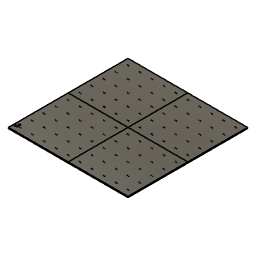
Base Plate (Autodesk Fusion 360 design; units mm, degrees)
Autodesk Fusion 360 part; units mm, degrees
note: some values were not read from the file. Chosen so that the rebuilt part matches the saved one: which face or edge a step refers to.
box "BoxPrimitive1" add length 175 width 175 height 3 placed x (0, 1, 0) y (-1, 0, 0) z (0, 0, 1) at (175, 0, 0) makes body 1
sketch "Sketch2" plane through (0, 0, 3) normal (0, 0, 1) x (-1, 0, 0)
  line L0 (-175, -175) -> (0, -175)
  line L1 (0, -175) -> (0, 0)
  line L2 (0, 0) -> (-175, 0)
  line L3 (-175, 0) -> (-175, -175)
  line L4 (0, 0) -> (-15.5, 0)
  line L5 (-15.5, 0) -> (-15.5, -17.5)
  line L6 (-15.5, -17.5) -> (0, -17.5)
  line L7 (0, -17.5) -> (0, 0)
  line L8 (-15.5, -17.5) -> (-19.5, -17.5)
  circle A0 centre (-19.5, -17.5) radius 0.425
  circle A1 centre (-15.5, -17.5) radius 0.425
  circle A2 centre (-50.5, -17.5) radius 0.425
  circle A3 centre (-54.5, -17.5) radius 0.425
  circle A4 centre (-85.5, -17.5) radius 0.425
  circle A5 centre (-89.5, -17.5) radius 0.425
  circle A6 centre (-120.5, -17.5) radius 0.425
  circle A7 centre (-124.5, -17.5) radius 0.425
  circle A8 centre (-155.5, -17.5) radius 0.425
  circle A9 centre (-159.5, -17.5) radius 0.425
  circle A10 centre (-15.5, -52.5) radius 0.425
  circle A11 centre (-19.5, -52.5) radius 0.425
  circle A12 centre (-50.5, -52.5) radius 0.425
  circle A13 centre (-54.5, -52.5) radius 0.425
  circle A14 centre (-85.5, -52.5) radius 0.425
  circle A15 centre (-89.5, -52.5) radius 0.425
  circle A16 centre (-120.5, -52.5) radius 0.425
  circle A17 centre (-124.5, -52.5) radius 0.425
  circle A18 centre (-155.5, -52.5) radius 0.425
  circle A19 centre (-159.5, -52.5) radius 0.425
  circle A20 centre (-15.5, -87.5) radius 0.425
  circle A21 centre (-19.5, -87.5) radius 0.425
  circle A22 centre (-50.5, -87.5) radius 0.425
  circle A23 centre (-54.5, -87.5) radius 0.425
  circle A24 centre (-85.5, -87.5) radius 0.425
  circle A25 centre (-89.5, -87.5) radius 0.425
  circle A26 centre (-120.5, -87.5) radius 0.425
  circle A27 centre (-124.5, -87.5) radius 0.425
  circle A28 centre (-155.5, -87.5) radius 0.425
  circle A29 centre (-159.5, -87.5) radius 0.425
  circle A30 centre (-15.5, -122.5) radius 0.425
  circle A31 centre (-19.5, -122.5) radius 0.425
  circle A32 centre (-50.5, -122.5) radius 0.425
  circle A33 centre (-54.5, -122.5) radius 0.425
  circle A34 centre (-85.5, -122.5) radius 0.425
  circle A35 centre (-89.5, -122.5) radius 0.425
  circle A36 centre (-120.5, -122.5) radius 0.425
  circle A37 centre (-124.5, -122.5) radius 0.425
  circle A38 centre (-155.5, -122.5) radius 0.425
  circle A39 centre (-159.5, -122.5) radius 0.425
  circle A40 centre (-15.5, -157.5) radius 0.425
  circle A41 centre (-19.5, -157.5) radius 0.425
  circle A42 centre (-50.5, -157.5) radius 0.425
  circle A43 centre (-54.5, -157.5) radius 0.425
  circle A44 centre (-85.5, -157.5) radius 0.425
  circle A45 centre (-89.5, -157.5) radius 0.425
  circle A46 centre (-120.5, -157.5) radius 0.425
  circle A47 centre (-124.5, -157.5) radius 0.425
  circle A48 centre (-155.5, -157.5) radius 0.425
  circle A49 centre (-159.5, -157.5) radius 0.425
  dimension "d6" = 15.5
  dimension "d7" = 17.5
  dimension "d8" = 4
  dimension "d9" = 0.85
  dimension "d10" = 0.85
  dimension "d13" = -35
  dimension "d14" = -35
  constraint horizontal L4
  constraint vertical L5
  constraint horizontal L6
  constraint vertical L7
  constraint coincident L1.end L2.start
  constraint perpendicular L5 L8
  constraint coincident L8.end A0.centre
  constraint coincident L5.end L6.start
  measures "d6" distance of L1.end L4.end
  measures "d7" distance of L1.end L6.end
  measures "d8" distance of L5.end L8.end
  measures "d9" diameter of A0
  measures "d10" diameter of A1
hole "Hole1" at (89.5, 157.5, 3) at (159.5, 157.5, 3) at (85.5, 157.5, 3) at (19.5, 157.5, 3) at (50.5, 157.5, 3) at (54.5, 157.5, 3) at (120.5, 157.5, 3) at (124.5, 157.5, 3) at (155.5, 157.5, 3) at (15.5, 157.5, 3) at (89.5, 122.5, 3) at (19.5, 52.5, 3) at (120.5, 87.5, 3) at (15.5, 52.5, 3) at (19.5, 87.5, 3) at (120.5, 122.5, 3) at (50.5, 87.5, 3) at (124.5, 87.5, 3) at (15.5, 122.5, 3) at (89.5, 52.5, 3) at (155.5, 52.5, 3) at (124.5, 122.5, 3) at (50.5, 52.5, 3) at (124.5, 52.5, 3) at (120.5, 52.5, 3) at (19.5, 122.5, 3) at (155.5, 87.5, 3) at (89.5, 87.5, 3) at (159.5, 52.5, 3) at (159.5, 122.5, 3) at (85.5, 87.5, 3) at (54.5, 122.5, 3) at (15.5, 87.5, 3) at (50.5, 122.5, 3) at (155.5, 122.5, 3) at (54.5, 52.5, 3) at (85.5, 52.5, 3) at (159.5, 87.5, 3) at (85.5, 122.5, 3) at (54.5, 87.5, 3) at (85.5, 17.5, 3) at (50.5, 17.5, 3) at (120.5, 17.5, 3) at (159.5, 17.5, 3) at (155.5, 17.5, 3) at (124.5, 17.5, 3) at (54.5, 17.5, 3) at (89.5, 17.5, 3) at (19.5, 17.5, 3) at (19.5, 17.5, 3) at (15.5, 17.5, 3) at (15.5, 17.5, 3) direction (0, 0, -1) diameter 1.1 depth 2.4 tip angle 180 countersink diameter 1.5 countersink angle 40 bodies 1
mirror "Mirror1" about plane through (175, 0, 0) normal (1, 0, 0) of bodies 1 makes body 2
mirror "Mirror2" about plane through (175, 0, 0) normal (0, -1, 0) of bodies 1 2 makes body 3 at (58.3333, -58.3333, 0) makes body 4 at (291.6667, -58.3333, 0)
sketch "Sketch3" plane through (0, 0, 3) normal (0, 0, 1) x (-1, 0, 0)
  circle A0 centre (-54.5, 17.5) radius 0.75
  circle A1 centre (-155.5, 17.5) radius 0.75
  circle A2 centre (-120.5, 17.5) radius 0.75
  circle A3 centre (-85.5, 17.5) radius 0.75
  circle A4 centre (-85.5, 122.5) radius 0.75
  circle A5 centre (-85.5, 52.5) radius 0.75
  circle A6 centre (-155.5, 122.5) radius 0.75
  circle A7 centre (-15.5, 87.5) radius 0.75
  circle A8 centre (-85.5, 87.5) radius 0.75
  circle A9 centre (-159.5, 52.5) radius 0.75
  circle A10 centre (-155.5, 87.5) radius 0.75
  circle A11 centre (-120.5, 52.5) radius 0.75
  circle A12 centre (-50.5, 52.5) radius 0.75
  circle A13 centre (-155.5, 52.5) radius 0.75
  circle A14 centre (-15.5, 122.5) radius 0.75
  circle A15 centre (-50.5, 87.5) radius 0.75
  circle A16 centre (-19.5, 87.5) radius 0.75
  circle A17 centre (-120.5, 87.5) radius 0.75
  circle A18 centre (-89.5, 122.5) radius 0.75
  circle A19 centre (-155.5, 157.5) radius 0.75
  circle A20 centre (-120.5, 157.5) radius 0.75
  circle A21 centre (-50.5, 157.5) radius 0.75
  circle A22 centre (-85.5, 157.5) radius 0.75
  circle A23 centre (-89.5, 157.5) radius 0.75
  circle A24 centre (-159.5, 157.5) radius 0.75
  circle A25 centre (-19.5, 157.5) radius 0.75
  circle A26 centre (-54.5, 157.5) radius 0.75
  circle A27 centre (-124.5, 157.5) radius 0.75
  circle A28 centre (-15.5, 157.5) radius 0.75
  circle A29 centre (-19.5, 52.5) radius 0.75
  circle A30 centre (-15.5, 52.5) radius 0.75
  circle A31 centre (-120.5, 122.5) radius 0.75
  circle A32 centre (-124.5, 87.5) radius 0.75
  circle A33 centre (-89.5, 52.5) radius 0.75
  circle A34 centre (-124.5, 122.5) radius 0.75
  circle A35 centre (-124.5, 52.5) radius 0.75
  circle A36 centre (-19.5, 122.5) radius 0.75
  circle A37 centre (-89.5, 87.5) radius 0.75
  circle A38 centre (-159.5, 122.5) radius 0.75
  circle A39 centre (-54.5, 122.5) radius 0.75
  circle A40 centre (-50.5, 122.5) radius 0.75
  circle A41 centre (-54.5, 52.5) radius 0.75
  circle A42 centre (-159.5, 87.5) radius 0.75
  circle A43 centre (-54.5, 87.5) radius 0.75
  circle A44 centre (-50.5, 17.5) radius 0.75
  circle A45 centre (-159.5, 17.5) radius 0.75
  circle A46 centre (-124.5, 17.5) radius 0.75
  circle A47 centre (-89.5, 17.5) radius 0.75
  circle A48 centre (-19.5, 17.5) radius 0.75
  circle A49 centre (-15.5, 17.5) radius 0.75
  line L0 (0, 175) -> (-175, 175)
  line L1 (-175, 175) -> (-175, 0)
  line L2 (-175, 0) -> (0, 0)
  line L3 (0, 0) -> (0, 175)
  line L4 (-15.5, 157.5) -> (-11.5, 157.5)
  line L5 (-11.5, 157.5) -> (-11.5, 161.5)
  line L6 (-11.5, 161.5) -> (-15.5, 161.5)
  line L7 (-15.5, 161.5) -> (-15.5, 157.5)
  line L8 (-11.5, 161.5) -> (-15.5, 161.5)
  line L9 (-15.5, 161.5) -> (-15.5, 165.5)
  line L10 (-15.5, 165.5) -> (-11.5, 165.5)
  line L11 (-11.5, 165.5) -> (-11.5, 161.5)
  line L12 (-11.5, 165.5) -> (-7.5, 165.5)
  line L13 (-7.5, 165.5) -> (-7.5, 161.5)
  line L14 (-7.5, 161.5) -> (-11.5, 161.5)
  line L15 (-11.5, 161.5) -> (-11.5, 165.5)
  line L16 (-11.5, 161.5) -> (-7.5, 161.5)
  line L17 (-7.5, 161.5) -> (-7.5, 157.5)
  line L18 (-7.5, 157.5) -> (-11.5, 157.5)
  line L19 (-11.5, 157.5) -> (-11.5, 161.5)
  line L20 (-11.5, 157.5) -> (-7.5, 157.5)
  line L21 (-7.5, 157.5) -> (-7.5, 153.5)
  line L22 (-7.5, 153.5) -> (-11.5, 153.5)
  line L23 (-11.5, 153.5) -> (-11.5, 157.5)
  line L24 (-7.5, 153.5) -> (-3.5, 153.5)
  line L25 (-3.5, 153.5) -> (-3.5, 157.5)
  line L26 (-3.5, 157.5) -> (-7.5, 157.5)
  line L27 (-7.5, 157.5) -> (-7.5, 153.5)
  line L28 (-7.5, 157.5) -> (-3.5, 157.5)
  line L29 (-3.5, 157.5) -> (-3.5, 161.5)
  line L30 (-3.5, 161.5) -> (-7.5, 161.5)
  line L31 (-7.5, 161.5) -> (-7.5, 157.5)
  line L32 (-7.5, 161.5) -> (-3.5, 161.5)
  line L33 (-3.5, 161.5) -> (-3.5, 165.5)
  line L34 (-3.5, 165.5) -> (-7.5, 165.5)
  line L35 (-7.5, 165.5) -> (-7.5, 161.5)
  line L36 (-15.5, 165.5) -> (-11.5, 165.5)
  line L37 (-11.5, 165.5) -> (-11.5, 169.5)
  line L38 (-11.5, 169.5) -> (-15.5, 169.5)
  line L39 (-15.5, 169.5) -> (-15.5, 165.5)
  line L40 (-11.5, 169.5) -> (-7.5, 169.5)
  line L41 (-7.5, 169.5) -> (-7.5, 165.5)
  line L42 (-7.5, 165.5) -> (-11.5, 165.5)
  line L43 (-11.5, 165.5) -> (-11.5, 169.5)
  line L44 (-7.5, 169.5) -> (-3.5, 169.5)
  line L45 (-3.5, 169.5) -> (-3.5, 165.5)
  line L46 (-3.5, 165.5) -> (-7.5, 165.5)
  line L47 (-7.5, 165.5) -> (-7.5, 169.5)
  line L48 (-15.5, 157.5) -> (-11.5, 157.5)
  line L49 (-11.5, 157.5) -> (-11.5, 153.5)
  line L50 (-11.5, 153.5) -> (-15.5, 153.5)
  line L51 (-15.5, 153.5) -> (-15.5, 157.5)
  line L52 (-15.5, 153.5) -> (-11.5, 153.5)
  line L53 (-11.5, 153.5) -> (-11.5, 149.5)
  line L54 (-11.5, 149.5) -> (-15.5, 149.5)
  line L55 (-15.5, 149.5) -> (-15.5, 153.5)
  line L56 (-11.5, 149.5) -> (-7.5, 149.5)
  line L57 (-7.5, 149.5) -> (-7.5, 153.5)
  line L58 (-7.5, 153.5) -> (-11.5, 153.5)
  line L59 (-11.5, 153.5) -> (-11.5, 149.5)
  line L60 (-7.5, 149.5) -> (-3.5, 149.5)
  line L61 (-3.5, 149.5) -> (-3.5, 153.5)
  line L62 (-3.5, 153.5) -> (-7.5, 153.5)
  line L63 (-7.5, 153.5) -> (-7.5, 149.5)
  line L64 (-15.5, 149.5) -> (-11.5, 149.5)
  line L65 (-11.5, 149.5) -> (-11.5, 145.5)
  line L66 (-11.5, 145.5) -> (-15.5, 145.5)
  line L67 (-15.5, 145.5) -> (-15.5, 149.5)
  line L68 (-11.5, 145.5) -> (-7.5, 145.5)
  line L69 (-7.5, 145.5) -> (-7.5, 149.5)
  line L70 (-7.5, 149.5) -> (-11.5, 149.5)
  line L71 (-11.5, 149.5) -> (-11.5, 145.5)
  line L72 (-7.5, 145.5) -> (-3.5, 145.5)
  line L73 (-3.5, 145.5) -> (-3.5, 149.5)
  line L74 (-3.5, 149.5) -> (-7.5, 149.5)
  line L75 (-7.5, 149.5) -> (-7.5, 145.5)
  dimension "d26" = 4
  dimension "d27" = 4
  dimension "d28" = 4
  dimension "d29" = 4
  dimension "d30" = 4
  dimension "d31" = 4
  dimension "d32" = 4
  dimension "d33" = 4
  dimension "d34" = 4
  dimension "d35" = 4
  dimension "d36" = 4
  dimension "d37" = 4
  dimension "d38" = 4
  dimension "d39" = 4
  dimension "d40" = 4
  dimension "d41" = 4
  dimension "d42" = 4
  dimension "d43" = 4
  dimension "d44" = 4
  dimension "d45" = 4
  dimension "d46" = 4
  dimension "d47" = 4
  constraint horizontal L4
  constraint vertical L5
  constraint horizontal L6
  constraint vertical L7
  constraint coincident A28.centre L4.start
  constraint horizontal L8
  constraint vertical L9
  constraint horizontal L10
  constraint vertical L11
  constraint horizontal L12
  constraint vertical L13
  constraint horizontal L14
  constraint vertical L15
  constraint horizontal L16
  constraint vertical L17
  constraint horizontal L18
  constraint vertical L19
  constraint horizontal L20
  constraint vertical L21
  constraint horizontal L22
  constraint vertical L23
  constraint horizontal L24
  constraint vertical L25
  constraint horizontal L26
  constraint vertical L27
  constraint horizontal L28
  constraint vertical L29
  constraint horizontal L30
  constraint vertical L31
  constraint horizontal L32
  constraint vertical L33
  constraint horizontal L34
  constraint vertical L35
  constraint horizontal L36
  constraint vertical L37
  constraint horizontal L38
  constraint vertical L39
  constraint horizontal L40
  constraint vertical L41
  constraint horizontal L42
  constraint vertical L43
  constraint horizontal L44
  constraint vertical L45
  constraint horizontal L46
  constraint vertical L47
  constraint horizontal L48
  constraint vertical L49
  constraint horizontal L50
  constraint vertical L51
  constraint horizontal L52
  constraint vertical L53
  constraint horizontal L54
  constraint vertical L55
  constraint horizontal L56
  constraint vertical L57
  constraint horizontal L58
  constraint vertical L59
  constraint horizontal L60
  constraint vertical L61
  constraint horizontal L62
  constraint vertical L63
  constraint horizontal L64
  constraint vertical L65
  constraint horizontal L66
  constraint vertical L67
  constraint horizontal L68
  constraint vertical L69
  constraint horizontal L70
  constraint vertical L71
  constraint horizontal L72
  constraint vertical L73
  constraint horizontal L74
  constraint vertical L75
  measures "d26" distance of A28.centre L4.end
  measures "d27" distance of A28.centre L6.end
  measures "d28" distance of L5.end L6.end
  measures "d29" distance of L5.end L10.end
  measures "d30" distance of L10.end L12.end
  measures "d31" distance of L10.end L5.end
  measures "d32" distance of L5.end L13.end
  measures "d33" distance of L5.end L4.end
  measures "d34" distance of L4.end L17.end
  measures "d35" distance of L4.end L22.end
  measures "d36" distance of L21.end L24.end
  measures "d37" distance of L21.end L17.end
  measures "d38" distance of L17.end L25.end
  measures "d39" distance of L17.end L13.end
  measures "d40" distance of L13.end L29.end
  measures "d41" distance of L13.end L12.end
  measures "d42" distance of L9.end L10.end
  measures "d43" distance of L9.end L38.end
  measures "d44" distance of L50.end L22.end
  measures "d45" distance of L50.end L54.end
  measures "d46" distance of L54.end L53.end
  measures "d47" distance of L54.end L66.end
hole "Hole2" at (11.5, -157.5, 3) at (11.5, -153.5, 3) at (11.5, -149.5, 3) at (11.5, -161.5, 3) at (7.5, -161.5, 3) at (7.5, -157.5, 3) at (7.5, -153.5, 3) at (7.5, -149.5, 3) at (3.5, -157.5, 3) at (3.5, -161.5, 3) direction (0, 0, -1) diameter 1.1 depth 2.4 tip angle 180 countersink diameter 1.5 countersink angle 40 bodies 3
move_face "OffsetFaces1" offset -0.2 4 faces at (350, -58.3333, 1) (291.6667, -175, 1) (0, -58.3333, 1) (58.3333, -175, 1) on bodies 3 4
move_face "OffsetFaces2" offset -0.2 2 faces at (350, 58.3333, 1) (291.6667, 175, 1) on bodies 2
extrude "Extrude2" cut 1 faces at (58.3333, 175, 1) along direction (0, -1, 0) blind 0.2 on bodies 1 bodies 1
extrude "Extrude3" cut 1 faces at (0, 58.2667, 1) along direction (1, 0, 0) blind 0.2 on bodies 1 bodies 1
equation "d7 = ( 35 / 2 ) * 1 mm"
